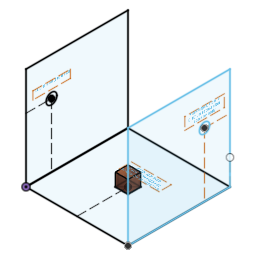
Final Design_ (1) (Autodesk Fusion 360 archive; units mm, degrees)
design "ManuPro2024_FinalProject_A_ (1)"
Autodesk Fusion 360 part; units mm, degrees
sketch "Sketch1" plane through (0, 0, 0) normal (0, 0, 1) x (1, 0, 0)
  line L0 (0, 0) -> (101.6, 0)
  line L1 (101.6, 0) -> (101.6, 101.6)
  line L2 (101.6, 101.6) -> (0, 101.6)
  line L3 (0, 101.6) -> (0, 0)
  line L4 (50.8, 0) -> (50.8, 50.8) construction
  line L5 (57.15, 57.15) -> (44.45, 57.15)
  line L6 (44.45, 57.15) -> (44.45, 44.45)
  line L7 (44.45, 44.45) -> (57.15, 44.45)
  line L8 (57.15, 44.45) -> (57.15, 57.15)
  line L9 (57.15, 57.15) -> (44.45, 44.45) construction
  line L10 (44.45, 57.15) -> (57.15, 44.45) construction
  line L11 (31.0753, 74.0973) -> (70.4547, 74.0973) construction
  line L12 (70.4547, 74.0973) -> (70.4547, 62.0849) construction
  line L13 (70.4547, 62.0849) -> (31.0753, 62.0849) construction
  line L14 (31.0753, 62.0849) -> (31.0753, 74.0973) construction
  point P0 (50.8, 50.8)
  dimension "d1" = 101.6
  dimension "d2" = 101.6
  dimension "d3" = 50.8
  dimension "d4" = 12.7
  dimension "d5" = 12.7
  dimension "d6" = 2.54
  constraint horizontal L0
  constraint vertical L1
  constraint horizontal L2
  constraint vertical L3
  constraint coincident L0.start L3.end
  constraint midpoint L0 L4.start
  constraint perpendicular L0 L4
  constraint horizontal L5
  constraint perpendicular L5 L6
  constraint parallel L5 L7
  constraint parallel L6 L8
  constraint coincident L9 P0
  constraint coincident L10 P0
  constraint coincident P0 L4.end
  measures "d1" distance of L0.start L0.end
  measures "d2" distance of L0.start L2.end
  measures "d3" distance of L4.start P0
  measures "d4" distance of L6.end L7.end
  measures "d5" distance of L5.end L6.end
sketch "Sketch2" plane through (0, 0, 0) normal (0, 0, 1) x (1, 0, 0)
sketch "Sketch3" plane through (0, 0, 0) normal (1, 0, 0) x (0, 1, 0)
  line L0 (0, 0) -> (101.6, 0)
  line L1 (101.6, 0) -> (101.6, 101.6)
  line L2 (101.6, 101.6) -> (0, 101.6)
  line L3 (0, 101.6) -> (0, 0)
  circle A0 centre (25.4, 63.5) radius 5.334
  line L4 (44.1613, 71.5131) -> (6.879, 71.5131) construction
  line L5 (6.879, 71.5131) -> (6.879, 79.4179) construction
  line L6 (6.879, 79.4179) -> (44.1613, 79.4179) construction
  line L7 (44.1613, 79.4179) -> (44.1613, 71.5131) construction
  line L8 (0, 63.5) -> (25.4, 63.5) construction
  line L9 (25.4, 63.5) -> (25.4, 0) construction
  dimension "d7" = 101.6
  dimension "d8" = 101.6
  dimension "d10" = 10.668
  dimension "d11" = 2.54
  dimension "d22" = 25.4
  dimension "d24" = 63.5
  constraint horizontal L0
  constraint vertical L1
  constraint horizontal L2
  constraint vertical L3
  constraint coincident L0.start L3.end
  constraint coincident A0.centre L8.end
  constraint coincident L3 L8.start
  constraint coincident L0 L9.end
  constraint perpendicular L0 L9
  measures "d7" distance of L0.start L0.end
  measures "d8" distance of L0.start L2.end
  measures "d10" diameter of A0
  measures "d22" distance of A0.centre L8.start
  measures "d24" distance of A0.centre L9.end
ref_plane "WorkPlane1" through (101.6, 50.8, 50.8) normal (1, 0, 0) x (0, 1, 0)
sketch "Sketch4" plane through (101.6, 50.8, 50.8) normal (1, 0, 0) x (0, 1, 0)
  line L0 (-50.8, -50.8) -> (50.8, -50.8)
  line L1 (50.8, -50.8) -> (50.8, 50.8)
  line L2 (50.8, 50.8) -> (-50.8, 50.8)
  line L3 (-50.8, 50.8) -> (-50.8, -50.8)
  line L4 (50.8, -50.8) -> (50.8, -25.4) construction
  circle A0 centre (25.4, 12.7) radius 5.08
  line L5 (5.853, 20.4085) -> (45.1217, 20.4616) construction
  line L6 (45.1217, 20.4616) -> (45.1056, 32.3635) construction
  line L7 (45.1056, 32.3635) -> (5.8369, 32.3104) construction
  line L8 (5.8369, 32.3104) -> (5.853, 20.4085) construction
  line L9 (25.4, 12.7) -> (50.8, 12.7) construction
  line L10 (25.4, 12.7) -> (25.4, -50.8) construction
  point P0 (-50.8, -50.8)
  dimension "d13" = 101.6
  dimension "d14" = 101.6
  dimension "d17" = 10.16
  dimension "d18" = 2.54
  dimension "d25" = 63.5
  dimension "d26" = 25.4
  constraint horizontal L0
  constraint vertical L1
  constraint horizontal L2
  constraint vertical L3
  constraint coincident P0 L0.start
  constraint perpendicular L0 L4
  constraint coincident A0.centre L9.start
  constraint coincident L1 L9.end
  constraint perpendicular L1 L9
  constraint coincident L0 L10.end
  constraint perpendicular L0 L10
  measures "d13" distance of P0 L0.end
  measures "d14" distance of P0 L2.end
  measures "d17" diameter of A0
  measures "d25" distance of A0.centre L10.end
  measures "d26" distance of A0.centre L9.end
extrude "Extrude1" add sketch "Sketch1" along normal blind 12.7 contours L5 L6 L7 L8
named bodies: "DEADZONE, DO NOT REMOVE"
